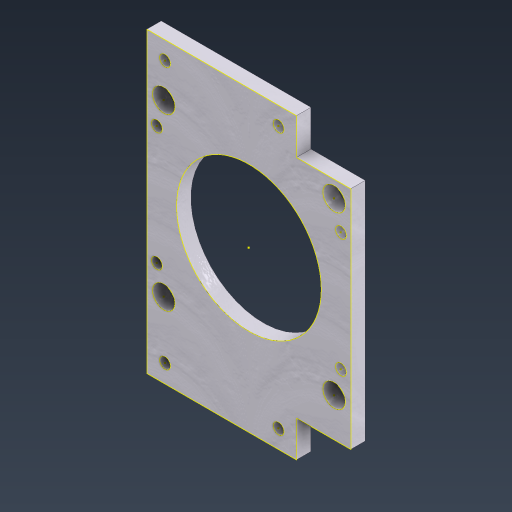
# Autodesk Inventor part: MotorHolder_3D
Saved by Autodesk Inventor 2023 (Build 270158000, 158)
## iProperties
Created: 2024-02-10
Part Number: MotorHolder_3D
Material: Aluminum 6061, Welded
Document SubType Name: Modeling
Designer: victo
Density: 2.7 g/cm^3
Appearance: Weld - Aluminum
Author: victo
Autodesk Inventor part; units mm, degrees
ref_plane "YZ Plane" through (0, 0, 0) normal (1, 0, 0) x (0, 1, 0)
ref_plane "XZ Plane" through (0, 0, 0) normal (0, 1, 0) x (-1, 0, 0)
ref_plane "XY Plane" through (0, 0, 0) normal (0, 0, 1) x (1, 0, 0)
sketch "Sketch1" plane through (0, 0, 0) normal (0, 0, 1) x (1, 0, 0)
  line L0 (-28.2, 28.2) -> (28.2, 28.2)
  line L1 (28.2, 28.2) -> (28.2, -28.2)
  line L2 (28.2, -28.2) -> (-28.2, -28.2)
  line L3 (-28.2, -28.2) -> (-28.2, 28.2)
  line L4 (-28.2, 28.2) -> (28.2, -28.2) construction
  line L5 (28.2, 28.2) -> (-28.2, -28.2) construction
  circle A0 centre (25.45, 16.4) radius 1.5
  circle A1 centre (25.45, -16.4) radius 1.5
  line L6 (0, 0) -> (0, 28.2) construction
  circle A2 centre (-25.45, 16.4) radius 1.5
  circle A3 centre (-25.45, -16.4) radius 1.5
  circle A4 centre (23.55, 23.55) radius 3.1
  circle A5 centre (-23.55, 23.55) radius 3.1
  circle A6 centre (-23.55, -23.55) radius 3.1
  circle A7 centre (23.55, -23.55) radius 3.1
  circle A8 centre (0, 0) radius 20
  line L7 (-28.2, 28.2) -> (13.2, 28.2)
  line L8 (13.2, 28.2) -> (13.2, 38.2)
  line L9 (13.2, 38.2) -> (-28.2, 38.2)
  line L10 (-28.2, 38.2) -> (-28.2, 28.2)
  circle A9 centre (-23.2, 33.2) radius 1.5
  circle A10 centre (8.2, 33.2) radius 1.5
  line L11 (13.2, -28.2) -> (-28.2, -28.2)
  line L12 (-28.2, -28.2) -> (-28.2, -44.2)
  line L13 (-28.2, -44.2) -> (13.2, -44.2)
  line L14 (13.2, -44.2) -> (13.2, -28.2)
  circle A11 centre (-23.2, -39.2) radius 1.5
  circle A12 centre (8.2, -39.2) radius 1.5
  line L15 (28.2, -28.2) -> (13.2, -28.2)
  line L16 (13.2, -28.2) -> (13.2, -34.2)
  line L17 (13.2, -34.2) -> (28.2, -34.2)
  line L18 (28.2, -34.2) -> (28.2, -28.2)
  point P0 (-28.2, -28.2)
  dimension "d0" = 3
  dimension "d1" = 56.4
  dimension "d2" = 16.4
  dimension "d3" = 25.45
  dimension "d4" = 56.4
  dimension "d5" = 3
  dimension "d6" = 16.4
  dimension "d7" = 25.45
  dimension "d8" = 6.2
  dimension "d9" = 23.55
  dimension "d10" = 23.55
  dimension "d13" = 360
  dimension "d17" = 40
  dimension "d18" = 10
  dimension "d19" = 15
  dimension "d20" = 3
  dimension "d21" = 3
  dimension "d22" = 5
  dimension "d23" = 5
  dimension "d24" = 5
  dimension "d25" = 5
  dimension "d26" = 16
  dimension "d27" = 15
  dimension "d28" = 0
  dimension "d29" = 3
  dimension "d30" = 3
  dimension "d31" = 5
  dimension "d32" = 5
  dimension "d33" = 5
  dimension "d34" = 5
  dimension "d35" = 6
  constraints: 38 end point, 13 centre point, 8 parallel, 4 horizontal, 4 perpendicular, 3 midpoint, 2 point on line, 2 symmetric about line, 1 coincident, 11 other
  measures "d0" diameter of A0
  measures "d1" distance between parallel lines of L3 L1
  measures "d2" vertical distance of L6.start A0.centre
  measures "d3" horizontal distance of L6.start A0.centre
  measures "d4" distance between parallel lines of L2 L0
  measures "d5" diameter of A1
  measures "d6" vertical distance of L6.start A1.centre
  measures "d7" horizontal distance of L6.start A1.centre
  measures "d8" diameter of A4
  measures "d9" horizontal distance of A4.centre L6.start
  measures "d10" horizontal distance of L6.start A4.centre
  measures "d17" diameter of A8
  measures "d18" distance between parallel lines of L0 L9
  measures "d19" distance between parallel lines of L1 L8
  measures "d20" diameter of A9
  measures "d21" diameter of A10
  measures "d22" distance from line of L8 A10.centre
  measures "d23" distance from line of L0 A10.centre
  measures "d24" distance from line of L7 A9.centre
  measures "d25" distance from line of L10 A9.centre
  measures "d26" distance of L12.end L11.end
  measures "d27" distance between parallel lines of L14 L1
  measures "d28" distance between parallel lines of L3 L12
  measures "d29" diameter of A11
  measures "d30" diameter of A12
  measures "d31" distance from line of A12.centre L13
  measures "d32" distance from line of L13 A11.centre
  measures "d33" distance from line of L12 A11.centre
  measures "d34" distance from line of L14 A12.centre
  measures "d35" distance of L16.end L15.end
extrude "Extrusion1" add sketch "Sketch1" along normal blind 4
sketch "Sketch3" plane through (0, 0, 4) normal (0, 0, 1) x (1, 0, 0)
  line L0 (28.2, -34.2) -> (28.2, 28.2) projected
  line L1 (28.2, 28.2) -> (13.2, 28.2) projected
  line L2 (13.2, 28.2) -> (13.2, 38.2) projected
  line L3 (13.2, 38.2) -> (-28.2, 38.2) projected
  line L4 (-28.2, 38.2) -> (-28.2, -44.2) projected
  line L5 (-28.2, -44.2) -> (13.2, -44.2) projected
  line L6 (13.2, -44.2) -> (13.2, -34.2) projected
  line L7 (13.2, -34.2) -> (28.2, -34.2) projected
  circle A0 centre (0, 0) radius 20 projected
  circle A1 centre (25.45, 16.4) radius 1.5 projected
  circle A2 centre (25.45, -16.4) radius 1.5 projected
  circle A3 centre (-25.45, 16.4) radius 1.5 projected
  circle A4 centre (-25.45, -16.4) radius 1.5 projected
  circle A5 centre (23.55, 23.55) radius 3.1 projected
  circle A6 centre (-23.55, 23.55) radius 3.1 projected
  circle A7 centre (-23.55, -23.55) radius 3.1 projected
  circle A8 centre (23.55, -23.55) radius 3.1 projected
  circle A9 centre (-23.2, 33.2) radius 1.5 projected
  circle A10 centre (8.2, 33.2) radius 1.5 projected
  circle A11 centre (-23.2, -39.2) radius 1.5 projected
  circle A12 centre (8.2, -39.2) radius 1.5 projected
equation "\"d4\" = d1"
equation "\"d6\" = d2"
equation "\"d7\" = d3"
body "Solid1"
